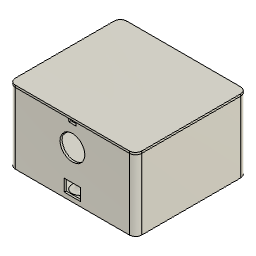
Enclosure (Autodesk Fusion 360 design; units mm, degrees)
Autodesk Fusion 360 part; units mm, degrees
note: some values were not read from the file. Set by a fixed rule: which face or edge a step refers to.
sketch "Sketch1" plane through (0, 0, 0) normal (0, 0, 1) x (1, 0, 0) in component "Case"
  line L0 (0, 0) -> (125, 0)
  line L1 (125, 0) -> (125, 110)
  line L2 (125, 110) -> (0, 110)
  line L3 (0, 110) -> (0, 0)
  dimension "d6" = 125
  dimension "d7" = 110
  constraint horizontal L0
  constraint vertical L1
  constraint horizontal L2
  constraint vertical L3
  constraint coincident L0.start L3.end
  measures "d6" distance of L0.start L0.end
  measures "d7" distance of L0.start L2.end
extrude "Extrude1" add sketch "Sketch1" along normal blind 70 makes body 1 in component "Case"
fillet "Fillet1" radius 6 4 edges at (125, 0, 35) (0, 0, 35) (125, 110, 35) (0, 110, 35) on bodies 1 in component "Case"
shell "Shell1" thickness 2 removed faces 1 at (81.3333, 36.6667, 70) on bodies 1 in component "Case"
sketch "Sketch2" plane through (2, 0, 0) normal (1, 0, 0) x (0, 1, 0) in component "Case"
  line L0 (104, 2) -> (104, 70)
  line L1 (104, 70) -> (6, 70)
  line L2 (6, 70) -> (6, 2)
  line L3 (6, 2) -> (104, 2)
  line L4 (27.5, 70) -> (82.5, 70)
  line L5 (82.5, 70) -> (82.5, 66)
  line L6 (82.5, 66) -> (27.5, 66)
  line L7 (27.5, 66) -> (27.5, 70)
  line L8 (55, 70) -> (55, 66) construction
  dimension "d13" = 4
  dimension "d14" = 55
  constraint horizontal L4
  constraint vertical L5
  constraint horizontal L6
  constraint vertical L7
  constraint coincident L1 L4.start
  constraint midpoint L1 L8.start
  constraint midpoint L6 L8.end
  constraint vertical L8
  measures "d13" distance of L4.start L6.end
  measures "d14" distance of L5.end L6.end
extrude "Extrude2" add sketch "Sketch2" along normal blind 6 draft -45 contours L1 L4 L5 L6 L7 bodies 1 in component "Case"
ref_plane "WorkPlane1" through (62.5, 55, 35) normal (-1, 0, 0) x (0, -1, 0) in component "Case"
mirror "Mirror1" about plane through (62.5, 55, 35) normal (-1, 0, 0) of "Extrude2" in component "Case"
sketch "Sketch1 (2)" plane through (0, 0, 70) normal (0, 0, 1) x (-1, 0, 0) in component "Cover"
  arc A0 (-2, -6) -> (-6, -2) centre (-6, -6) ccw
  line L0 (-2, -6) -> (-2, -27.5)
  line L1 (-2, -27.5) -> (-2, -82.5)
  line L2 (-2, -82.5) -> (-2, -104)
  arc A1 (-6, -108) -> (-2, -104) centre (-6, -104) ccw
  line L3 (-6, -108) -> (-119, -108)
  arc A2 (-123, -104) -> (-119, -108) centre (-119, -104) ccw
  line L4 (-123, -104) -> (-123, -82.5)
  line L5 (-123, -82.5) -> (-123, -27.5)
  line L6 (-123, -27.5) -> (-123, -6)
  arc A3 (-119, -2) -> (-123, -6) centre (-119, -6) ccw
  line L7 (-119, -2) -> (-6, -2)
  arc A4 (-6, -110) -> (0, -104) centre (-6, -104) ccw
  line L8 (0, -104) -> (0, -6)
  arc A5 (0, -6) -> (-6, 0) centre (-6, -6) ccw
  line L9 (-6, 0) -> (-119, 0)
  arc A6 (-119, 0) -> (-125, -6) centre (-119, -6) ccw
  line L10 (-125, -6) -> (-125, -104)
  arc A7 (-125, -104) -> (-119, -110) centre (-119, -104) ccw
  line L11 (-119, -110) -> (-6, -110)
extrude "Extrude1'" add sketch "Sketch1 (2)" along normal blind 2 separate body contours A0 L0 L1 L2 A1 L3 A2 L4 L5 L6 A3 L7 | A4 L8 A5 L9 A6 L10 A7 L11 makes body 2 in component "Cover"
sketch "Sketch2 (2)" plane through (0, 0, 70) normal (0, 0, -1) x (1, 0, 0) in component "Cover"
  line L0 (6, -110) -> (119, -110)
  arc A0 (119, -110) -> (125, -104) centre (119, -104) ccw
  line L1 (125, -104) -> (125, -6)
  arc A1 (125, -6) -> (119, 0) centre (119, -6) ccw
  line L2 (119, 0) -> (6, 0)
  arc A2 (6, 0) -> (0, -6) centre (6, -6) ccw
  line L3 (0, -6) -> (0, -104)
  arc A3 (0, -104) -> (6, -110) centre (6, -104) ccw
  arc A4 (2.2, -104) -> (6, -107.8) centre (6, -104) ccw
  line L4 (6, -107.8) -> (119, -107.8)
  arc A5 (119, -107.8) -> (122.8, -104) centre (119, -104) ccw
  line L5 (122.8, -104) -> (122.8, -6)
  arc A6 (122.8, -6) -> (119, -2.2) centre (119, -6) ccw
  line L6 (119, -2.2) -> (6, -2.2)
  arc A7 (6, -2.2) -> (2.2, -6) centre (6, -6) ccw
  line L7 (2.2, -6) -> (2.2, -104)
extrude "Extrude2'" add sketch "Sketch2 (2)" along normal blind 4 contours A4 L4 A5 L5 A6 L6 A7 L7 bodies 2 in component "Cover"
extrude "Extrude3" cut sketch "Sketch2" along normal blind 4 draft -45 from surface at 0.2 contours L1 L4 L5 L6 L7 bodies 2 in component "Cover"
mirror "Mirror1'" about plane through (62.5, 55, 35) normal (-1, 0, 0) of "Extrude3" in component "Cover"
shell "Shell1'" thickness 2 removed faces 1 at (42.4, 45.8333, 66) on bodies 2 in component "Cover"
chamfer "Chamfer1" distance 0.6 angle 45 1 edges at (122.8, 55, 66) on bodies 2 in component "Cover"
chamfer "Chamfer2" distance 0.6 angle 45 1 edges at (2.2, 55, 66) on bodies 2 in component "Cover"
sketch "Sketch3" plane through (0, 2, 0) normal (0, 1, 0) x (-1, 0, 0) in component "Case"
  line L0 (-6, 2) -> (-6, 70)
  line L1 (-6, 70) -> (-119, 70)
  line L2 (-119, 70) -> (-119, 2)
  line L3 (-119, 2) -> (-6, 2)
  line L4 (-70.5, 2) -> (-54.5, 2)
  line L5 (-54.5, 2) -> (-54.5, 16.5)
  line L6 (-54.5, 16.5) -> (-70.5, 16.5)
  line L7 (-70.5, 16.5) -> (-70.5, 2)
  line L8 (-62.5, 2) -> (-62.5, 16.5) construction
  line L9 (-70.5, 4.5) -> (-54.5, 4.5)
  dimension "d39" = 14.5
  dimension "d40" = 16
  constraint horizontal L4
  constraint vertical L5
  constraint horizontal L6
  constraint vertical L7
  constraint coincident L3 L4.start
  constraint midpoint L3 L8.start
  constraint midpoint L6 L8.end
  constraint vertical L8
  measures "d39" distance of L4.start L6.end
  measures "d40" distance of L5.end L6.end
extrude "Extrude3'" cut sketch "Sketch3" against normal up to surface (2 mm away) contours L5 L6 L7 L9 bodies 1 in component "Case"
sketch "Sketch4" plane through (0, 0, 0) normal (0, -1, 0) x (1, 0, 0) in component "Case"
  line L0 (54.5, 16.5) -> (70.5, 16.5)
  line L1 (70.5, 16.5) -> (70.5, 4.5)
  line L2 (54.5, 4.5) -> (54.5, 16.5)
  line L3 (6, 70) -> (6, 0)
  line L4 (6, 0) -> (119, 0)
  line L5 (119, 0) -> (119, 70)
  line L6 (119, 70) -> (6, 70)
  circle A0 centre (62.5, 46.625) radius 12.25
  line L7 (62.5, 70) -> (62.5, 46.625) construction
  line L8 (70.5, 4.5) -> (54.5, 4.5)
  dimension "d48" = 24.5
  dimension "d49" = 23.375
  constraint midpoint L6 L7.start
  constraint coincident A0.centre L7.end
  constraint vertical L7
  measures "d48" diameter of A0
  measures "d49" distance of L7.start A0.centre
extrude "Extrude4" cut sketch "Sketch4" against normal up to surface (2 mm away) contours A0 bodies 1 in component "Case"
sketch "Sketch5" plane through (0, 110, 0) normal (0, 1, 0) x (-1, 0, 0) in component "Case"
  line L0 (-6, 0) -> (-6, 70)
  line L1 (-6, 70) -> (-119, 70)
  line L2 (-119, 70) -> (-119, 0)
  line L3 (-119, 0) -> (-6, 0)
  line L4 (-85.385, 60) -> (-39.615, 60)
  line L5 (-15.625, 36.01) -> (-15.625, 35.99)
  line L6 (-39.615, 12) -> (-85.385, 12)
  line L7 (-109.375, 35.99) -> (-109.375, 36.01)
  arc A0 (-85.385, 60) -> (-109.375, 36.01) centre (-85.385, 36.01) ccw
  arc A1 (-15.625, 36.01) -> (-39.615, 60) centre (-39.615, 36.01) ccw
  arc A2 (-39.615, 12) -> (-15.625, 35.99) centre (-39.615, 35.99) ccw
  arc A3 (-109.375, 35.99) -> (-85.385, 12) centre (-85.385, 35.99) ccw
  line L8 (-102.3485, 52.9735) -> (-22.6515, 19.0265) construction
  line L9 (-22.6515, 52.9735) -> (-102.3485, 19.0265) construction
  line L10 (-62.5, 70) -> (-62.5, 36)
  point P0 (-109.375, 60)
  point P1 (-15.625, 60)
  point P2 (-109.375, 12)
  dimension "d61" = 48
  dimension "d62" = 93.75
  dimension "d63" = 23.99
  dimension "d64" = 23.99
  dimension "d65" = 23.99
  dimension "d66" = 23.99
  dimension "d68" = 34
  constraint horizontal L4
  constraint vertical L5
  constraint horizontal L6
  constraint vertical L7
  constraint coincident P0 L4
  constraint coincident P0 L7
  constraint tangent L4 A0
  constraint tangent L7 A0
  constraint coincident P1 L4
  constraint coincident P1 L5
  constraint tangent L4 A1
  constraint tangent L5 A1
  constraint tangent L5 A2
  constraint tangent L6 A2
  constraint coincident P2 L6
  constraint coincident P2 L7
  constraint tangent L6 A3
  constraint tangent L7 A3
  constraint midpoint A0 L8.start
  constraint midpoint A2 L8.end
  constraint midpoint A1 L9.start
  constraint midpoint A3 L9.end
  constraint midpoint L1 L10.start
  constraint midpoint L8 L10.end
  constraint vertical L10
  measures "d61" distance of P0 P2
  measures "d62" distance of P0 P1
  measures "d63" radius of A0
  measures "d64" radius of A1
  measures "d65" radius of A2
  measures "d66" radius of A3
  measures "d68" distance of L10.start L10.end
extrude "Extrude5" cut sketch "Sketch5" against normal up to surface (2 mm away) contours L4 L5 L6 L7 A0 A1 A2 A3 bodies 1 in component "Case"
sketch "Sketch6" plane through (0, 0, 0) normal (0, -1, 0) x (1, 0, 0) in component "Case"
  circle A0 centre (62.5, 46.625) radius 12.25
  line L0 (54.5, 16.5) -> (70.5, 16.5)
  line L1 (70.5, 16.5) -> (70.5, 4.5)
  line L2 (54.5, 4.5) -> (54.5, 16.5)
  line L3 (6, 70) -> (6, 0)
  line L4 (6, 0) -> (119, 0)
  line L5 (119, 0) -> (119, 70)
  line L6 (119, 70) -> (6, 70)
  line L7 (66.05, 70) -> (58.95, 70)
  line L8 (58.95, 70) -> (58.95, 67)
  line L9 (58.95, 67) -> (66.05, 67)
  line L10 (66.05, 67) -> (66.05, 70)
  line L11 (62.5, 70) -> (62.5, 67) construction
  line L12 (70.5, 4.5) -> (54.5, 4.5)
  dimension "d72" = 3
  dimension "d73" = 7.1
  constraint horizontal L7
  constraint vertical L8
  constraint horizontal L9
  constraint vertical L10
  constraint coincident L6 L7.start
  constraint midpoint L6 L11.start
  constraint midpoint L9 L11.end
  constraint vertical L11
  measures "d72" distance of L7.start L9.end
  measures "d73" distance of L8.end L9.end
extrude "Extrude6" cut sketch "Sketch6" against normal up to surface (2 mm away) contours L6 L7 L8 L9 L10 bodies 1 in component "Case"
sketch "Sketch3 (2)" plane through (0, 2.2, 0) normal (0, -1, 0) x (1, 0, 0) in component "Cover"
  line L0 (119, 70) -> (6, 70)
  line L1 (6, 70) -> (6, 66)
  line L2 (6, 66) -> (119, 66)
  line L3 (119, 66) -> (119, 70)
  line L4 (66.05, 66) -> (58.95, 66)
  line L5 (58.95, 66) -> (58.95, 70)
  line L6 (58.95, 70) -> (66.05, 70)
  line L7 (66.05, 70) -> (66.05, 66)
  line L8 (62.5, 66) -> (62.5, 70)
  dimension "d76" = 4
  dimension "d77" = 7.1
  constraint horizontal L4
  constraint vertical L5
  constraint horizontal L6
  constraint vertical L7
  constraint coincident L2 L4.start
  constraint midpoint L2 L8.start
  constraint midpoint L6 L8.end
  constraint vertical L8
  measures "d76" distance of L4.start L6.end
  measures "d77" distance of L5.end L6.end
extrude "Extrude4'" cut sketch "Sketch3 (2)" against normal up to surface (2 mm away) contours L0 L2 L4 L6 L7 L8 | L0 L2 L4 L5 L6 L8 bodies 2 in component "Cover"
sketch "Sketch7" plane through (0, 0, 2) normal (0, 0, 1) x (-1, 0, 0) in component "Case"
  arc A0 (-6, -108) -> (-2, -104) centre (-6, -104) ccw
  line L0 (-2, -104) -> (-2, -6)
  arc A1 (-2, -6) -> (-6, -2) centre (-6, -6) ccw
  line L1 (-6, -2) -> (-119, -2)
  arc A2 (-119, -2) -> (-123, -6) centre (-119, -6) ccw
  line L2 (-123, -6) -> (-123, -104)
  arc A3 (-123, -104) -> (-119, -108) centre (-119, -104) ccw
  line L3 (-119, -108) -> (-6, -108)
  line L4 (-52.8, -108) -> (-52.8, -102.68)
  line L5 (-52.8, -102.68) -> (-55.55, -102.68)
  line L6 (-55.55, -102.68) -> (-55.55, -100.68)
  line L7 (-55.55, -100.68) -> (-50.8, -100.68)
  line L8 (-50.8, -100.68) -> (-50.8, -108)
  line L9 (-50.8, -108) -> (-52.8, -108)
  line L10 (-72.2, -108) -> (-72.2, -102.68)
  line L11 (-72.2, -102.68) -> (-69.45, -102.68)
  line L12 (-69.45, -102.68) -> (-69.45, -100.68)
  line L13 (-69.45, -100.68) -> (-74.2, -100.68)
  line L14 (-74.2, -100.68) -> (-74.2, -108)
  line L15 (-72.2, -108) -> (-74.2, -108)
  line L16 (-52.8, -105.34) -> (-72.2, -105.34) construction
  line L17 (-62.5, -105.34) -> (-62.5, -108) construction
  dimension "d81" = 2
  dimension "d86" = 2
  dimension "d88" = 19.4
  dimension "d90" = 4.75
  dimension "d91" = 4.75
  dimension "d94" = 5.32
  dimension "d95" = 2
  dimension "d96" = 5.32
  dimension "d97" = 2
  constraint coincident L3 L4.start
  constraint perpendicular L3 L4
  constraint perpendicular L4 L5
  constraint perpendicular L5 L6
  constraint perpendicular L6 L7
  constraint coincident L3 L8.end
  constraint perpendicular L3 L8
  constraint coincident L3 L10.start
  constraint perpendicular L3 L10
  constraint perpendicular L10 L11
  constraint perpendicular L11 L12
  constraint perpendicular L12 L13
  constraint coincident L3 L14.end
  constraint perpendicular L3 L14
  constraint midpoint L4 L16.start
  constraint midpoint L10 L16.end
  constraint midpoint L16 L17.start
  constraint midpoint L3 L17.end
  constraint vertical L17
  measures "d81" distance of L4.start L8.end
  measures "d86" distance of L10.start L14.end
  measures "d88" horizontal distance of L16.start L16.end
  measures "d90" distance of L6.end L7.end
  measures "d91" distance of L12.end L13.end
  measures "d94" distance of L10.start L10.end
  measures "d95" distance of L11.end L12.end
  measures "d96" distance of L4.start L4.end
  measures "d97" distance of L5.end L6.end
extrude "Extrude7" add sketch "Sketch7" along normal blind 10 contours L3 L4 L5 L6 L7 L8 L9 | L3 L10 L11 L12 L13 L14 L15 bodies 1 in component "Case"
sketch "Sketch9" plane through (2, 0, 0) normal (1, 0, 0) x (0, 1, 0) in component "Case"
  line L0 (82.5, 70) -> (82.5, 66)
  line L1 (82.5, 66) -> (27.5, 66)
  line L2 (27.5, 66) -> (27.5, 70)
  line L3 (27.5, 70) -> (6, 70)
  line L4 (6, 70) -> (6, 2)
  line L5 (6, 2) -> (104, 2)
  line L6 (104, 2) -> (104, 70)
  line L7 (104, 70) -> (82.5, 70)
  circle A0 centre (44.84, 42.35) radius 1.25
  circle A1 centre (65.16, 42.35) radius 1.25
  circle A2 centre (65.16, 29.65) radius 1.27
  circle A3 centre (44.84, 29.65) radius 1.27
  circle A4 centre (44.84, 42.35) radius 0.85
  circle A5 centre (65.16, 42.35) radius 0.85
  circle A6 centre (44.84, 29.65) radius 0.87
  circle A7 centre (65.16, 29.65) radius 0.87
  dimension "d116" = -0.4
  dimension "d117" = -0.4
  dimension "d118" = -0.4
  dimension "d119" = -0.4
extrude "Extrude9" add sketch "Sketch9" along normal blind 12 contours A4 | A5 | A6 | A7 bodies 1 in component "Case"
sketch "Sketch10" plane through (123, 0, 0) normal (-1, 0, 0) x (0, -1, 0) in component "Case"
  line L0 (-82.5, 66) -> (-82.5, 70)
  line L1 (-82.5, 70) -> (-104, 70)
  line L2 (-104, 70) -> (-104, 2)
  line L3 (-104, 2) -> (-6, 2)
  line L4 (-6, 2) -> (-6, 70)
  line L5 (-6, 70) -> (-27.5, 70)
  line L6 (-27.5, 70) -> (-27.5, 66)
  line L7 (-27.5, 66) -> (-82.5, 66)
  circle A0 centre (-65.16, 42.35) radius 1.25
  circle A1 centre (-44.84, 42.35) radius 1.25
  circle A2 centre (-44.84, 29.65) radius 1.25
  circle A3 centre (-65.16, 29.65) radius 1.25
  circle A4 centre (-65.16, 42.35) radius 0.85
  circle A5 centre (-44.84, 42.35) radius 0.85
  circle A6 centre (-65.16, 29.65) radius 0.85
  circle A7 centre (-44.84, 29.65) radius 0.85
  dimension "d122" = -0.4
  dimension "d123" = -0.4
  dimension "d124" = -0.4
  dimension "d125" = -0.4
extrude "Extrude10" add sketch "Sketch10" along normal blind 12 contours A4 | A5 | A6 | A7 bodies 1 in component "Case"
sketch "Sketch11" plane through (52.8, 0, 0) normal (1, 0, 0) x (0, 1, 0) in component "Case"
  line L0 (102.68, 2) -> (108, 2)
  line L1 (108, 2) -> (108, 12)
  line L2 (108, 12) -> (102.68, 12)
  line L3 (102.68, 12) -> (102.68, 2)
  line L4 (108, 12) -> (105.8, 12)
  line L5 (105.8, 12) -> (105.8, 9.5)
  line L6 (105.8, 9.5) -> (108, 9.5)
  line L7 (108, 9.5) -> (108, 12)
  dimension "d139" = 2.2
  dimension "d140" = 2.5
  constraint horizontal L4
  constraint vertical L5
  constraint horizontal L6
  constraint vertical L7
  constraint coincident L1.end L2.start
  measures "d139" distance of L5.end L6.end
  measures "d140" distance of L4.end L5.end
extrude "Extrude11" cut sketch "Sketch11" along normal blind 2 from surface at -2 contours L1 L2 L4 L5 L6 L7 bodies 1 in component "Case"
mirror "Mirror2" about plane through (62.5, 55, 35) normal (-1, 0, 0) of "Extrude11" in component "Case"
sketch "Sketch12" plane through (0, 0, 2) normal (0, 0, 1) x (-1, 0, 0) in component "Case"
  line L0 (-74.2, -108) -> (-74.2, -100.68)
  line L1 (-74.2, -100.68) -> (-69.45, -100.68)
  line L2 (-69.45, -100.68) -> (-69.45, -102.68)
  line L3 (-69.45, -102.68) -> (-72.2, -102.68)
  line L4 (-72.2, -102.68) -> (-72.2, -108)
  line L5 (-72.2, -108) -> (-52.8, -108)
  line L6 (-52.8, -108) -> (-52.8, -102.68)
  line L7 (-52.8, -102.68) -> (-55.55, -102.68)
  line L8 (-55.55, -102.68) -> (-55.55, -100.68)
  line L9 (-55.55, -100.68) -> (-50.8, -100.68)
  line L10 (-50.8, -100.68) -> (-50.8, -108)
  line L11 (-50.8, -108) -> (-6, -108)
  arc A0 (-6, -108) -> (-2, -104) centre (-6, -104) ccw
  line L12 (-2, -104) -> (-2, -6)
  arc A1 (-2, -6) -> (-6, -2) centre (-6, -6) ccw
  line L13 (-6, -2) -> (-119, -2)
  arc A2 (-119, -2) -> (-123, -6) centre (-119, -6) ccw
  line L14 (-123, -6) -> (-123, -104)
  arc A3 (-123, -104) -> (-119, -108) centre (-119, -104) ccw
  line L15 (-119, -108) -> (-74.2, -108)
  circle A4 centre (-68.1, -13.05) radius 1.05
  circle A5 centre (-56.9, -13.05) radius 1.05
  circle A6 centre (-56.85, -60.1) radius 1.05
  circle A7 centre (-68.15, -60.1) radius 1.05
  circle A8 centre (-68.1, -13.05) radius 2.9
  circle A9 centre (-56.9, -13.05) radius 2.9
  circle A10 centre (-56.85, -60.1) radius 2.9
  circle A11 centre (-68.15, -60.1) radius 2.9
  dimension "d150" = 1.85
  dimension "d151" = 1.85
  dimension "d152" = 1.85
  dimension "d153" = 1.85
extrude "Extrude12" add sketch "Sketch12" along normal blind 6 contours A4 | A5 | A6 | A7 | A8 | A9 | A10 | A11 bodies 1 in component "Case"
sketch "Sketch13" plane through (0, 0, 8) normal (0, 0, 1) x (-1, 0, 0) in component "Case"
  circle A0 centre (-68.1, -13.05) radius 2.9
  circle A1 centre (-68.1, -13.05) radius 0.9
extrude "Extrude13" cut sketch "Sketch13" along normal blind 6 from surface at -6 contours A1 bodies 1 in component "Case"
sketch "Sketch14" plane through (0, 0, 8) normal (0, 0, 1) x (-1, 0, 0) in component "Case"
  circle A0 centre (-56.9, -13.05) radius 2.9
  circle A1 centre (-56.9, -13.05) radius 0.9
extrude "Extrude14" cut sketch "Sketch14" along normal blind 6 from surface at -6 contours A1 bodies 1 in component "Case"
sketch "Sketch15" plane through (0, 0, 8) normal (0, 0, 1) x (-1, 0, 0) in component "Case"
  circle A0 centre (-68.15, -60.1) radius 2.9
  circle A1 centre (-68.15, -60.1) radius 0.9
extrude "Extrude15" cut sketch "Sketch15" along normal blind 6 from surface at -6 contours A1 bodies 1 in component "Case"
sketch "Sketch16" plane through (0, 0, 8) normal (0, 0, 1) x (-1, 0, 0) in component "Case"
  circle A0 centre (-56.85, -60.1) radius 2.9
  circle A1 centre (-56.85, -60.1) radius 0.9
extrude "Extrude16" cut sketch "Sketch16" along normal blind 6 from surface at -6 contours A1 bodies 1 in component "Case"
fillet "Fillet3" radius 5 4 edges at (70.8037, 12.0013, 2) (59.6037, 12.0013, 2) (70.8537, 59.0513, 2) (59.5537, 59.0513, 2) on bodies 1 in component "Case"
sketch "Sketch17" plane through (0, 2, 0) normal (0, 1, 0) x (-1, 0, 0) in component "Case"
  line L0 (-58.95, 70) -> (-58.95, 67)
  line L1 (-58.95, 67) -> (-66.05, 67)
  line L2 (-66.05, 67) -> (-66.05, 70)
  line L3 (-66.05, 70) -> (-119, 70)
  line L4 (-119, 70) -> (-119, 2)
  line L5 (-119, 2) -> (-6, 2)
  line L6 (-6, 2) -> (-6, 70)
  line L7 (-6, 70) -> (-58.95, 70)
  line L8 (-70.5, 4.5) -> (-70.5, 16.5)
  line L9 (-70.5, 16.5) -> (-54.5, 16.5)
  line L10 (-54.5, 16.5) -> (-54.5, 4.5)
  line L11 (-54.5, 4.5) -> (-70.5, 4.5)
  circle A0 centre (-62.5, 46.625) radius 12.25
  circle A1 centre (-86.24, 29.65) radius 1.25
  circle A2 centre (-86.24, 42.35) radius 1.25
  circle A3 centre (-106.56, 42.35) radius 1.25
  circle A4 centre (-106.56, 29.65) radius 1.25
  circle A5 centre (-106.56, 42.35) radius 0.85
  circle A6 centre (-86.24, 42.35) radius 0.85
  circle A7 centre (-106.56, 29.65) radius 0.85
  circle A8 centre (-86.24, 29.65) radius 0.85
  dimension "d185" = -0.4
  dimension "d186" = -0.4
  dimension "d187" = -0.4
  dimension "d188" = -0.4
extrude "Extrude17" add sketch "Sketch17" along normal blind 12 contours A5 | A6 | A7 | A8 bodies 1 in component "Case"
component "Enclosure" placed x (1, 0, 0) y (0, 1, 0) z (0, 0, 1) at (0, 0, 0)
component "Case" placed x (1, 0, 0) y (0, 1, 0) z (0, 0, 1) at (0, 0, 0) in component "Enclosure"
component "Cover" placed x (1, 0, 0) y (0, 1, 0) z (0, 0, 1) at (0, 0, 0) in component "Enclosure"
equation "width = 110 mm"
equation "length = 125 mm"
equation "height = 70 mm"
equation "wall = 2 mm"
equation "clearance = 0.2 mm"
equation "d6 = length"
equation "d7 = width"
equation "d8 = height"
equation "d12 = wall"
equation "d13 = wall * 2"
equation "d14 = width / 2"
equation "d19 = wall"
equation "d21 = -( wall + clearance )"
equation "d22 = wall * 2"
equation "d25 = wall * 2"
equation "d29 = wall"
equation "pico_gap = 9 mm"
equation "usb_width = 16 mm"
equation "usb_height = 12 mm"
equation "d39 = usb_height + usb_offset"
equation "d40 = usb_width"
equation "button_width = 24.5 mm"
equation "d48 = button_width"
equation "d49 = ( ( height - usb_height - wall - ( button_width / 2 ) ) + opener_height ) / 2"
equation "opener_height = 3 mm"
equation "d61 = height - wall - ( ltr_offset * 2 )"
equation "d62 = length * 0.75"
equation "d63 = ( ( height - wall - ( ltr_offset * 2 ) ) / 2 ) - 0.01 mm"
equation "d64 = ( ( height - wall - ( ltr_offset * 2 ) ) / 2 ) - 0.01 mm"
equation "d65 = ( ( height - wall - ( ltr_offset * 2 ) ) / 2 ) - 0.01 mm"
equation "d66 = ( ( height - wall - ( ltr_offset * 2 ) ) / 2 ) - 0.01 mm"
equation "ltr_offset = 10 mm"
equation "d68 = ( height - wall ) / 2"
equation "opener_width = 7.1 mm"
equation "d72 = opener_height"
equation "d73 = opener_width"
equation "d76 = wall * 2"
equation "d77 = opener_width"
equation "d81 = wall"
equation "ltr_length = 19 mm"
equation "ltr_width = 5.12 mm"
equation "d86 = wall"
equation "d88 = ltr_length + ( clearance * 2 )"
equation "ltr_header_width = 13.1 mm"
equation "d90 = ( ( ltr_length - ltr_header_width ) / 2 ) + wall - clearance"
equation "d91 = ( ( ltr_length - ltr_header_width ) / 2 ) + wall - clearance"
equation "d94 = ltr_width + clearance"
equation "d95 = wall"
equation "d96 = ltr_width + clearance"
equation "d97 = wall"
equation "d98 = ltr_offset"
equation "pin_height = 12 mm"
equation "d116 = side_pin_offset"
equation "d117 = side_pin_offset"
equation "d118 = side_pin_offset"
equation "d119 = side_pin_offset"
equation "d120 = pin_height"
equation "d122 = side_pin_offset"
equation "d123 = side_pin_offset"
equation "d124 = side_pin_offset"
equation "d125 = side_pin_offset"
equation "d126 = pin_height"
equation "side_pin_offset = -0.4 mm"
equation "pin_fillet = 4 mm"
equation "mesh_width = 2 mm + clearance"
equation "d139 = mesh_width"
equation "d140 = ltr_offset * 0.25"
equation "d142 = wall"
equation "screw_diameter = 2 mm"
equation "screw_height = 6 mm"
equation "screw_clearance = 0.2 mm"
equation "screw_wall = screw_diameter"
equation "d150 = ( ( screw_diameter - screw_clearance ) + 2 * screw_wall - 2.1 mm ) / 2"
equation "d151 = ( ( screw_diameter - screw_clearance ) + 2 * screw_wall - 2.1 mm ) / 2"
equation "d152 = ( ( screw_diameter - screw_clearance ) + 2 * screw_wall - 2.1 mm ) / 2"
equation "d153 = ( ( screw_diameter - screw_clearance ) + 2 * screw_wall - 2.1 mm ) / 2"
equation "d154 = screw_height"
equation "d157 = -screw_wall"
equation "d159 = screw_height"
equation "d161 = -screw_wall"
equation "d163 = screw_height"
equation "d165 = -screw_wall"
equation "d167 = screw_height"
equation "d169 = -screw_wall"
equation "d171 = screw_height"
equation "d174 = screw_height - 1 mm"
equation "usb_offset = 2.5 mm"
equation "d176 = -usb_offset"
equation "d178 = ( length - ( 2 * 6 ) * 1 mm ) * 1 / 5"
equation "d185 = side_pin_offset"
equation "d186 = side_pin_offset"
equation "d187 = side_pin_offset"
equation "d188 = side_pin_offset"
equation "d189 = pin_height"
